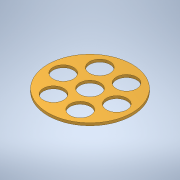
# Autodesk Inventor part: separator
Saved by Autodesk Inventor 2022 (Build 260153000, 153)
## iProperties
Created: 2021-07-22
Part Number: separator
Material: Generic
Document SubType Name: Modeling
Designer: WASHINGTON
Density: 1 g/cm^3
Appearance: Brass - Satin
Author: WASHINGTON
Autodesk Inventor part; units mm, degrees
ref_plane "YZ Plane" through (0, 0, 0) normal (1, 0, 0) x (0, 1, 0)
ref_plane "XZ Plane" through (0, 0, 0) normal (0, 1, 0) x (-1, 0, 0)
ref_plane "XY Plane" through (0, 0, 0) normal (0, 0, 1) x (1, 0, 0)
sketch "Sketch3" plane through (0, 0, 0) normal (0, 1, 0) x (-1, 0, 0)
  circle A0 centre (0, 0) radius 33
  circle A1 centre (0, 0) radius 8
  line L0 (0, 0) -> (32, 0) construction
  line L1 (0, 0) -> (34, 0) construction
  line L2 (24.0416, -24.0416) -> (20.5061, -20.5061)
  line L3 (0, 0) -> (34, 0) construction
  line L4 (0, 0) -> (22.2739, 0)
  line L5 (0, 0) -> (21, 0)
  circle A2 centre (21, 0) radius 8
  circle A3 centre (10.5, 18.1865) radius 8
  circle A4 centre (-10.5, 18.1865) radius 8
  circle A5 centre (-21, 0) radius 8
  circle A6 centre (-10.5, -18.1865) radius 8
  circle A7 centre (10.5, -18.1865) radius 8
  dimension "d15" = 66
  dimension "d17" = 16
  dimension "d25" = 34
  dimension "d27" = 5
  dimension "d31" = 21
  dimension "d32" = 16
  dimension "d35" = 360
  constraints: 12 end point, 8 centre point, 3 horizontal, 2 coincident, 2 point on line, 13 other
  measures "d15" diameter of A0
  measures "d17" diameter of A1
  measures "d25" distance of L0.start L2.start
  measures "d27" distance of L2.start L2.end
  measures "d31" distance of L0.start L5.end
  measures "d32" diameter of A2
extrude "Extrusion1" add sketch "Sketch3" along normal blind 2
body "Solid2"
